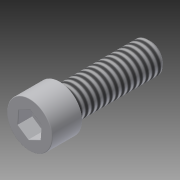
# Autodesk Inventor part: 4_40_hex_cap_screw
Saved by Autodesk Inventor 2014 (Build 180170000, 170)
## iProperties
Created: 2014-03-24
Part Number: 4_40_hex_cap_screw
Material: Generic
Document SubType Name: Modeling
Designer: stephenholtz
Density: 1 g/cm^3
Appearance: Default
Mass: 0.991884 g
Surface Area: 7.50729 cm^2
Volume: 0.991884 cm^3
Description: COTS
Author: stephenholtz
Autodesk Inventor part; units mm, degrees
ref_plane "YZ Plane" through (0, 0, 0) normal (1, 0, 0) x (0, 1, 0)
ref_plane "XZ Plane" through (0, 0, 0) normal (0, 1, 0) x (-1, 0, 0)
ref_plane "XY Plane" through (0, 0, 0) normal (0, 0, 1) x (1, 0, 0)
sketch "Sketch1" plane through (0, 0, 0) normal (0, 0, 1) x (1, 0, 0)
  circle A0 centre (0, 0) radius 4.7625
  dimension "max_head_dia" = 9.525
  constraints: 1 centre point, 1 coincident
  measures "max_head_dia" diameter of A0
extrude "Extrusion1" add sketch "Sketch1" along normal blind 6.35
sketch "Sketch2" plane through (0, 0, 0) normal (0, 0, -1) x (-1, 0, 0)
  circle A0 centre (0, 0) radius 4.7625 projected
  circle A1 centre (0, 0) radius 3.175
  dimension "max_body_dia" = 6.35
  constraints: 1 centre point, 1 coincident
  measures "max_body_dia" diameter of A1
extrude "Extrusion2" add sketch "Sketch2" along normal blind 19.05 contours A1
sketch "Sketch3" plane through (0, 0, 6.35) normal (0, 0, 1) x (1, 0, 0)
  circle A0 centre (0, 0) radius 4.7625 projected
  line L0 (-2.2794, 1.5378) -> (0.192, 2.7429)
  line L1 (0.192, 2.7429) -> (2.4715, 1.2051)
  line L2 (2.4715, 1.2051) -> (2.2794, -1.5378)
  line L3 (2.2794, -1.5378) -> (-0.192, -2.7429)
  line L4 (-0.192, -2.7429) -> (-2.4715, -1.2051)
  line L5 (-2.4715, -1.2051) -> (-2.2794, 1.5378)
  dimension "hex_socket_size" = 4.7625
  constraints: 12 end point, 1 coincident, 13 other
  measures "hex_socket_size" distance between parallel lines of L3 L0
extrude "Extrusion3" cut sketch "Sketch3" against normal blind 3.048 contours L0 L1 L2 L3 L4 L5
thread "Thread2" size "1/4-20 UNC" class "2A" standard "ANSI Unified Screw Threads" length 25.4
chamfer "Chamfer1" distance 0.635 angle 45 1 edges at (3.175, 0, -19.05)
fillet "Fillet1" radius 0.127 1 edges at (-4.7625, 0, 0)
fillet "Fillet2" radius 0.127 1 edges at (-4.7625, 0, 6.35)
fillet "Fillet3" radius 0.127 6 edges at (-1.3318, -1.974, 6.35) (-2.3754, 0.1663, 6.35) (-1.0437, 2.1403, 6.35) (1.3318, 1.974, 6.35) (2.3754, -0.1663, 6.35) (1.0437, -2.1403, 6.35)
body "Solid1"
